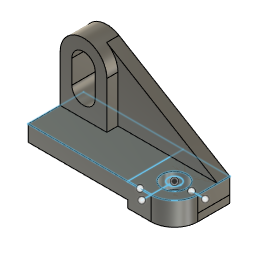
stage1finalblock (Autodesk Fusion 360 design; units mm, degrees)
Autodesk Fusion 360 part; units mm, degrees
note: some values were not read from the file. Set by a fixed rule: which sketch regions a step uses.
sketch "Sketch1" plane through (0, 0, 0) normal (0, 1, 0) x (1, 0, 0)
  line L0 (0, 0) -> (38, 0)
  line L1 (38, 0) -> (38, -38)
  line L2 (38, -38) -> (0, -38)
  line L3 (0, -38) -> (0, 0)
  circle A0 centre (19, -38) radius 19
  line L4 (9.5, -38) -> (28.5, -38)
  line L5 (28.5, -38) -> (28.5, -19)
  line L6 (28.5, -19) -> (9.5, -19)
  line L7 (9.5, -19) -> (9.5, -38)
  circle A1 centre (19, -38) radius 9.5
  circle A2 centre (19, -19) radius 9.5
  dimension "d1" = 38
  dimension "d2" = 38
  dimension "d3" = 19
  dimension "d4" = 19
  dimension "d5" = 19
  dimension "d6" = 9.5
  constraint horizontal L0
  constraint vertical L1
  constraint horizontal L2
  constraint vertical L3
  constraint coincident L0.start L3.end
  constraint coincident L1.end A0
  constraint tangent L1 A0
  constraint coincident L2.end A0
  constraint horizontal L4
  constraint vertical L5
  constraint horizontal L6
  constraint vertical L7
  constraint coincident L4.end A1
  constraint tangent L5 A1
  constraint coincident L4.start A1
  constraint coincident L5.end A2
  constraint tangent L5 A2
  constraint coincident L6.end A2
  measures "d1" distance of L0.start L0.end
  measures "d2" distance of L0.start L2.end
  measures "d3" distance of L4.start L4.end
  measures "d4" distance of L4.start L6.end
  measures "d5" distance of L0 L6
  measures "d6" distance of L3 L7
extrude "Extrude1" add sketch "Sketch1" along normal blind 19 contours L0 L1 L3 A0 L5 L7 A2 | L2 A0 L7 | L2 A0 A1 | L2 A0 L5 makes body 1
sketch "Sketch1 (2)" plane through (0, 19, 0) normal (0, 1, 0) x (-1, 0, 0) in component "sideline"
  arc A0 (-28.5, 19) -> (-9.5, 19) centre (-19, 19) ccw
  line L0 (-28.5, 19) -> (-28.5, 38)
  arc A1 (-9.5, 38) -> (-28.5, 38) centre (-19, 38) ccw
  line L1 (-9.5, 38) -> (-9.5, 19)
  arc A2 (0, 38) -> (-38, 38) centre (-19, 38) ccw
  line L2 (-38, 38) -> (-38, 0)
  line L3 (-38, 0) -> (0, 0)
  line L4 (0, 0) -> (0, 38)
  line L5 (-38, 0) -> (-119, 0)
  line L6 (-119, 0) -> (-28.7963, 54.2798)
  dimension "d9" = 81
  constraint coincident L2.end L3.start
  constraint perpendicular L2 L5
  constraint coincident A2 L6.end
  constraint tangent A2 L6
  measures "d9" distance of L2.end L5.end
extrude "Extrude1'" add sketch "Sketch1 (2)" against normal blind 10 separate body contours A2 L2 L5 L6 makes body 2 in component "sideline"
combine "Combine1" operation add target body 2 tool bodies 1 in component "sideline"
sketch "Sketch2" plane through (0, 0, 0) normal (0, 0, 1) x (1, 0, 0) in component "sideline"
  line L0 (119, 19) -> (0, 19)
  line L1 (0, 19) -> (0, -26)
  line L2 (0, -26) -> (100, -26)
  line L3 (119, -7) -> (119, 19)
  line L4 (113.8585, -7) -> (125, -7)
  circle A0 centre (100, -7) radius 10
  circle A1 centre (100, -7) radius 5
  arc A2 (100, -26) -> (119, -7) centre (100, -7) ccw
  line L5 (100, -7) -> (100, -33.6154)
  line L6 (100, -26) -> (91, -26)
  line L7 (100, -26) -> (81, -26)
  line L8 (81, -26) -> (81, 19)
  dimension "d19" = 19
  constraint horizontal L0
  constraint vertical L1
  constraint horizontal L2
  constraint vertical L3
  constraint perpendicular L3 L4
  constraint concentric A0 A2
  constraint concentric A1 A2
  constraint coincident L4 L3.start
  constraint coincident A0.centre A1.centre
  constraint perpendicular L2 L5
  constraint perpendicular L5 L6
  constraint parallel L2 L7
  constraint coincident L0 L8.end
  constraint perpendicular L0 L8
  measures "d19" distance of L2.end L7.end
extrude "Extrude2" add sketch "Sketch2" against normal blind 13 contours L0 L2 L3 A2 L6 L7 L8 | L0 L1 L2 L8 bodies 2 in component "sideline"
sketch "Sketch3" plane through (0, 0, -13) normal (0, 0, -1) x (1, 0, 0) in component "sideline"
  circle A0 centre (100, 7) radius 10
  line L0 (119, -19) -> (119, 7)
  arc A1 (119, 7) -> (100, 26) centre (100, 7) ccw
  line L1 (100, 26) -> (0, 26)
  line L2 (0, 26) -> (0, -19)
  line L3 (0, -19) -> (119, -19)
  circle A2 centre (100, 7) radius 5
  line L4 (80.9955, 26) -> (80.9955, -19)
  dimension "d22" = 10
  constraint concentric A0 A2
  constraint coincident L1 L4.start
  constraint coincident L3 L4.end
  constraint perpendicular L3 L4
  measures "d22" diameter of A2
extrude "Extrude3" add sketch "Sketch3" along normal blind 6 contours A0 | L0 A1 L1 L3 L4 bodies 2 in component "sideline"
component "sideline" placed x (1, 0, 0) y (0, 1, 0) z (0, 0, 1) at (0, 0, 0)
